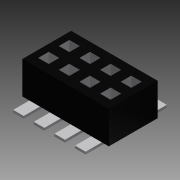
# Autodesk Inventor part: 127mm2Row8PosFemale
Saved by Autodesk Inventor 2014 (Build 180170000, 170)
## iProperties
Created: 2015-11-06
Part Number: 127mm2Row8PosFemale
Material: Generic
Document SubType Name: Modeling
Designer: Owner
Density: 1 g/cm^3
Appearance: Default
Author: Owner
Autodesk Inventor part; units mm, degrees
ref_plane "YZ Plane" through (0, 0, 0) normal (1, 0, 0) x (0, 1, 0)
ref_plane "XZ Plane" through (0, 0, 0) normal (0, 1, 0) x (-1, 0, 0)
ref_plane "XY Plane" through (0, 0, 0) normal (0, 0, 1) x (1, 0, 0)
sketch "Sketch1" plane through (0, 0, 0) normal (0, 1, 0) x (-1, 0, 0)
  line L0 (-2.5885, 2.7601) -> (2.7315, 2.7601)
  line L1 (2.7315, 2.7601) -> (2.7315, -0.2399)
  line L2 (2.7315, -0.2399) -> (-2.5885, -0.2399)
  line L3 (-2.5885, -0.2399) -> (-2.5885, 2.7601)
  point P0 (0, 0)
  dimension "d0" = 5.32
  dimension "d1" = 3
  constraints: 8 end point, 2 parallel, 1 horizontal, 1 perpendicular
  measures "d0" distance of L0.start L0.end
  measures "d1" distance of L0.end L1.end
extrude "Extrusion1" add sketch "Sketch1" along normal blind 2
sketch "Sketch2" plane through (0, 0, 0) normal (0, -1, 0) x (1, 0, 0)
  line L0 (-2.7315, 2.7601) -> (-2.7315, -0.2399) projected
  line L1 (-2.7315, -0.2399) -> (2.5885, -0.2399) projected
  line L2 (-2.3015, 3.7601) -> (-1.6515, 3.7601)
  line L3 (-1.6515, 3.7601) -> (-1.6515, -1.2399)
  line L4 (-1.6515, -1.2399) -> (-2.3015, -1.2399)
  line L5 (-2.3015, -1.2399) -> (-2.3015, 3.7601)
  point P0 (0, 0)
  dimension "d4" = 5
  dimension "d5" = 0.65
  dimension "d6" = 1
  dimension "d7" = 0.43
  constraints: 8 end point, 2 parallel, 1 horizontal, 1 perpendicular
  measures "d4" distance of L4.end L2.start
  measures "d5" distance of L3.end L4.end
  measures "d6" distance between parallel lines of L1 L4
  measures "d7" distance between parallel lines of L5 L0
extrude "Extrusion2" add sketch "Sketch2" along normal blind 0.15
pattern_linear "Rectangular Pattern1" count 4 spacing 1.27 along (1, 0, 0) of "Extrusion2"
sketch "Sketch3" plane through (0, 2, 0) normal (0, 1, 0) x (1, 0, 0)
  line L0 (2.5885, 0.2399) -> (-2.7315, 0.2399) projected
  line L1 (-2.7315, 0.2399) -> (-2.7315, -2.7601) projected
  line L2 (-2.3015, -0.3001) -> (-1.6515, -0.3001)
  line L3 (-1.6515, -0.3001) -> (-1.6515, -0.9501)
  line L4 (-1.6515, -0.9501) -> (-2.3015, -0.9501)
  line L5 (-2.3015, -0.9501) -> (-2.3015, -0.3001)
  point P0 (0, 0)
  dimension "d13" = 0.65
  dimension "d14" = 0.65
  dimension "d15" = 0.43
  dimension "d16" = 0.54
  constraints: 8 end point, 2 parallel, 1 horizontal, 1 perpendicular
  measures "d13" distance of L2.end L3.end
  measures "d14" distance of L3.end L4.end
  measures "d15" distance between parallel lines of L1 L5
  measures "d16" distance between parallel lines of L0 L2
extrude "Extrusion3" cut sketch "Sketch3" against normal through all
pattern_linear "Rectangular Pattern2" count 4 spacing 1.27 along (1, 0, 0) count 2 spacing 1.27 along (0, 0, 1) of "Extrusion3"
body "Solid1"
